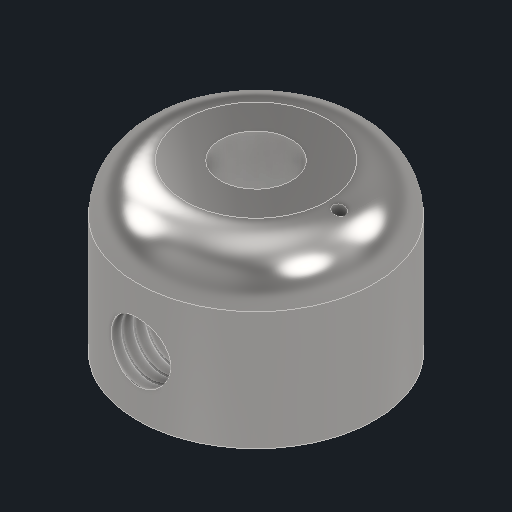
# Autodesk Inventor part: Lower Lock Cap
Saved by Autodesk Inventor 2027.1 (Build 311270010, 270A)
## iProperties
Created: 2025-09-16
Part Number: Lower Lock Cap
Material: Brass, Soft Yellow
Document SubType Name: Modeling
Designer: SD
Density: 8.47 g/cm^3
Appearance: Semi-Polished
Mass: 3.87264 g
Surface Area: 4.25052 cm^2
Volume: 0.457218 cm^3
Project: Automatic Tea Steeping mechanism
Length: 7.000 mm
BOM-Mass: 0.00359
BOM-Area: 0.000
Diameter: 10.000 mm
Procurement: Fabricate - 1st round
Build Stage: 1
Preferred Material: C36000 Brass
Author: SD
Title: Lower Lock Cap
Autodesk Inventor part; units mm, degrees
ref_plane "YZ Plane" through (0, 0, 0) normal (1, 0, 0) x (0, 1, 0)
ref_plane "XZ Plane" through (0, 0, 0) normal (0, 1, 0) x (-1, 0, 0)
ref_plane "XY Plane" through (0, 0, 0) normal (0, 0, 1) x (1, 0, 0)
sketch "Sketch1" plane through (0, 0, 0) normal (0, 1, 0) x (-1, 0, 0)
  circle A0 centre (0, 0) radius 5
  dimension "Diameter" = 10
  constraints: 1 centre point, 1 coincident
  measures "Diameter" diameter of A0
extrude "Extrusion1" add sketch "Sketch1" along normal mid plane 7
fillet "Fillet1" radius 2 1 edges at (5, 3.5, 0)
sketch "Sketch2" plane through (0, -3.5, 0) normal (0, -1, 0) x (1, 0, 0)
  circle A0 centre (0, 0) radius 1.5
  dimension "d4" = 3
  constraints: 1 centre point, 1 coincident
  measures "d4" diameter of A0
extrude "Extrusion2" cut sketch "Sketch2" against normal through all
sketch "Sketch3" plane through (0, 0, 0) normal (0, 0, 1) x (1, 0, 0)
  circle A0 centre (0, -1) radius 1.25
  line L0 (-5, -3.5) -> (5, -3.5) projected
  point P0 (0, 0)
  dimension "d7" = 2.5
  dimension "d8" = 2.5
  constraints: 1 centre point, 1 vertical alignment
  measures "d7" diameter of A0
  measures "d8" distance from line of A0.centre L0
extrude "Extrusion3" cut sketch "Sketch3" along normal blind 7
ref_plane "Work Plane1" through (0, 8.5, 0) normal (0, 1, 0) x (1, 0, 0)
sketch "Sketch4" plane through (0, 8.5, 0) normal (0, 1, 0) x (1, 0, 0)
  circle A0 centre (3.5, 0) radius 0.25
  point P0 (0, 0)
  dimension "d12" = 0.5
  dimension "d13" = 3.5
  constraints: 1 centre point, 1 horizontal alignment
  measures "d12" diameter of A0
  measures "d13" distance of point (0, 0) A0.centre
extrude "Extrusion4" cut sketch "Sketch4" against normal blind 9
thread "Thread1" size "M3x0.5" class "6H" standard "ANSI Metric M Profile" length 5
body "Solid1"
